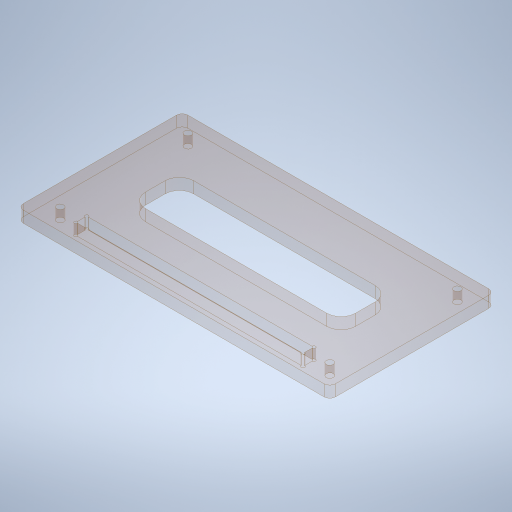
# Autodesk Inventor part: Marco conectores IC DC
Saved by Autodesk Inventor 2024.2 (Build 282272000, 272)
## iProperties
Created: 2024-09-17
Part Number: Marco conectores IC DC
Material: Polycarbonate, Smoke
Document SubType Name: Modeling
Designer: ja.restrepo1
Density: 1.2 g/cm^3
Appearance: Polycarbonate - Smoked
Author: ja.restrepo1
Autodesk Inventor part; units mm, degrees
ref_plane "YZ Plane" through (0, 0, 0) normal (1, 0, 0) x (0, 1, 0)
ref_plane "XZ Plane" through (0, 0, 0) normal (0, 1, 0) x (-1, 0, 0)
ref_plane "XY Plane" through (0, 0, 0) normal (0, 0, 1) x (1, 0, 0)
sketch "Sketch1" plane through (0, 0, 0) normal (0, 1, 0) x (-1, 0, 0)
  line L0 (55, -28) -> (-55, -28)
  line L1 (-55, -28) -> (-55, 28)
  line L2 (-55, 28) -> (55, 28) construction
  line L3 (55, 28) -> (55, -28)
  circle A0 centre (47.5, -22.5) radius 1.25
  circle A1 centre (-47.5, -22.5) radius 1.25
  circle A2 centre (-47.5, 22.5) radius 1.25
  circle A3 centre (47.5, 22.5) radius 1.25
  line L4 (47.5, -22.5) -> (-47.5, -22.5) construction
  line L5 (-47.5, -22.5) -> (-47.5, 22.5) construction
  line L6 (-32, -9) -> (32, -9)
  line L7 (32, 8) -> (-32, 8)
  line L8 (-55, 28) -> (-55, 30)
  line L9 (-55, 30) -> (55, 30)
  line L10 (55, 30) -> (55, 28)
  line L11 (37, 3) -> (37, -4)
  line L12 (-37, 3) -> (-37, -4)
  arc A4 (37, 3) -> (32, 8) centre (32, 3) ccw
  arc A5 (32, -9) -> (37, -4) centre (32, -4) ccw
  arc A6 (-32, 8) -> (-37, 3) centre (-32, 3) ccw
  arc A7 (-37, -4) -> (-32, -9) centre (-32, -4) ccw
  point P0 (0, 0)
  point P1 (-55, 0)
  point P2 (0, 28)
  point P3 (-47.5, 0)
  point P4 (0, -22.5)
  point P5 (-37, -9)
  point P6 (37, -9)
  point P7 (37, 8)
  point P8 (-37, 8)
  point P9 (0, 8)
  dimension "d0" = 110
  dimension "d1" = 56
  dimension "d2" = 2.5
  dimension "d3" = 95
  dimension "d4" = 45
  dimension "d18" = 2
  dimension "d20" = 74
  dimension "d21" = 19
  dimension "d22" = 17
  dimension "d23" = 5
  constraints: 26 end point, 8 centre point, 8 point on circle, 8 point on line, 8 tangent, 6 equal radius, 5 midpoint, 5 parallel, 5 vertical alignment, 4 horizontal alignment, 3 perpendicular, 2 horizontal, 2 vertical
  measures "d0" distance of L1.end L2.end
  measures "d1" distance of L0.end L1.end
  measures "d2" diameter of A0
  measures "d3" distance of L4.start L4.end
  measures "d4" distance of L4.end L5.end
  measures "d18" distance of L1.end L8.end
  measures "d20" distance of point (37, 8) point (-37, 8)
  measures "d21" distance between parallel lines of L0 L6
  measures "d22" distance between parallel lines of L6 L7
  measures "d23" radius of A4
extrude "Extrusion1" add sketch "Sketch1" along normal mid plane 4
fillet "Fillet1" radius 2 4 edges at (55, 0, -28) (-55, 0, -28) (-55, 0, 30) (55, 0, 30)
sketch "Sketch2" plane through (0, 2, 0) normal (0, 1, 0) x (1, 0, 0)
  line L0 (-40, -20.65) -> (-39.4, -20.65) construction
  line L1 (40, -20.65) -> (40, -21.25) construction
  line L2 (40, -24.45) -> (39.4, -24.45) construction
  line L3 (-40, -24.45) -> (-40, -23.85) construction
  arc A0 (-40, -23.85) -> (-39.4, -24.45) centre (-40, -24.45) ccw
  arc A1 (-39.4, -20.65) -> (-40, -21.25) centre (-40, -20.65) ccw
  arc A2 (40, -21.25) -> (39.4, -20.65) centre (40, -20.65) ccw
  arc A3 (39.4, -24.45) -> (40, -23.85) centre (40, -24.45) ccw
  line L4 (-40, -23.85) -> (-40, -21.25)
  line L5 (-39.4, -24.45) -> (-40, -24.45) construction
  arc A4 (-40, -21.25) -> (-39.4, -20.65) centre (-40, -20.65) ccw construction
  line L6 (-40, -21.25) -> (-40, -20.65) construction
  line L7 (-39.4, -20.65) -> (39.4, -20.65)
  line L8 (39.4, -24.45) -> (-39.4, -24.45)
  line L9 (40, -23.85) -> (40, -24.45) construction
  arc A5 (40, -23.85) -> (39.4, -24.45) centre (40, -24.45) ccw construction
  arc A6 (39.4, -20.65) -> (40, -21.25) centre (40, -20.65) ccw construction
  line L10 (40, -21.25) -> (40, -23.85)
  line L11 (39.4, -20.65) -> (40, -20.65) construction
  line L12 (-53, -30) -> (53, -30) projected
  point P0 (0, 0)
  point P1 (0, -24.45)
  dimension "d9" = 3.8
  dimension "d11" = 80
  dimension "d14" = 1.2
  dimension "d19" = 5.55
  constraints: 24 end point, 18 parallel, 14 point on circle, 9 perpendicular, 7 centre point, 4 coincident, 3 equal radius, 3 horizontal, 1 midpoint, 1 vertical alignment
  measures "d9" distance between parallel lines of L0 L2
  measures "d11" distance of L2.start L3.start
  measures "d14" diameter of A0
  measures "d19" distance between parallel lines of L12 L8
extrude "Extrusion2" cut sketch "Sketch2" against normal through all
body "Solid1"
